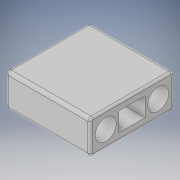
# Autodesk Inventor part: Y_Slider_Part_mit_Schrittmotor
Saved by Autodesk Inventor 2019 (Build 230136000, 136)
## iProperties
Created: 2018-08-19
Part Number: Y_Slider_Part_mit_Schrittmotor
Material: Generic
Document SubType Name: Modeling
Designer: Julia
Density: 1 g/cm^3
Appearance: Default
Author: Julia
Autodesk Inventor part; units mm, degrees
ref_plane "YZ Plane" through (0, 0, 0) normal (1, 0, 0) x (0, 1, 0)
ref_plane "XZ Plane" through (0, 0, 0) normal (0, 1, 0) x (-1, 0, 0)
ref_plane "XY Plane" through (0, 0, 0) normal (0, 0, 1) x (1, 0, 0)
sketch "Sketch1" plane through (0, 0, 0) normal (0, 1, 0) x (-1, 0, 0)
  line L0 (40, 40) -> (-40, 40)
  line L1 (-40, 40) -> (-40, -40)
  line L2 (-40, -40) -> (40, -40)
  line L3 (40, -40) -> (40, 40)
  point P0 (0, 0)
  point P1 (40, 0)
  point P2 (0, 40)
  dimension "d0" = 80
  dimension "d1" = 80
  constraints: 8 end point, 2 midpoint, 2 parallel, 1 horizontal, 1 horizontal alignment, 1 perpendicular, 1 vertical alignment
  measures "d0" distance of L2.end L0.start
  measures "d1" distance of L1.end L2.end
extrude "Extrusion1" add sketch "Sketch1" along normal blind 32
sketch "Sketch27" plane through (-40, 0, 40) normal (0, 0, 1) x (1, 0, 0)
  line L0 (20, 27) -> (60, 27)
  line L1 (60, 27) -> (60, 5)
  line L2 (60, 5) -> (20, 5)
  line L3 (20, 5) -> (20, 27)
  line L4 (0, 0) -> (80, 0) projected
  line L5 (0, 32) -> (80, 32) projected
  line L6 (0, 0) -> (0, 32) projected
  line L7 (80, 0) -> (80, 32) projected
  point P0 (40, 0)
  dimension "d171" = 5
  dimension "d172" = 5
  dimension "d173" = 20
  dimension "d174" = 20
  constraints: 8 end point, 2 parallel, 1 horizontal, 1 perpendicular
  measures "d171" distance between parallel lines of L4 L2
  measures "d172" distance between parallel lines of L5 L0
  measures "d173" distance between parallel lines of L6 L3
  measures "d174" distance between parallel lines of L7 L1
extrude "Extrusion21" cut sketch "Sketch27" against normal up to next contours L0 L1 L2 L3
sketch "Sketch28" plane through (-40, 0, -40) normal (-1, 0, 0) x (0, 0, 1)
  line L0 (0, 0) -> (0, 32) projected
  point P0 (40, 0)
  point P1 (15, 16)
  point P2 (65, 16)
  point P3 (0, 16)
  point P4 (0, 16)
  dimension "d177" = 25
  dimension "d178" = 25
  constraints: 2 horizontal alignment, 2 midpoint
  measures "d177" horizontal distance of point (40, 0) point (15, 16)
  measures "d178" horizontal distance of point (65, 16) point (40, 0)
hole "Hole8" at (-40, 16, -25) at (-40, 16, 25) direction (1, 0, 0) diameter 20 end through all
sketch "Sketch29" plane through (-40, 0, -40) normal (-1, 0, 0) x (0, 0, 1)
  line L0 (52.5, 25) -> (27.5, 25)
  line L1 (27.5, 25) -> (27.5, 7)
  line L2 (27.5, 7) -> (52.5, 7)
  line L3 (52.5, 7) -> (52.5, 25)
  line L4 (0, 32) -> (80, 32) projected
  line L5 (0, 0) -> (80, 0) projected
  point P0 (40, 0)
  point P1 (40, 7)
  point P2 (40, 0)
  dimension "d186" = 7
  dimension "d187" = 7
  dimension "d188" = 25
  constraints: 8 end point, 2 midpoint, 2 parallel, 1 horizontal, 1 perpendicular, 1 vertical alignment
  measures "d186" distance between parallel lines of L0 L4
  measures "d187" distance between parallel lines of L5 L2
  measures "d188" distance of L1.end L2.end
extrude "Extrusion22" cut sketch "Sketch29" against normal through all
extrude "Extrusion23" add sketch "Sketch27" against normal blind 4 contours L0 L1 L2 L3
sketch "Sketch30" plane through (40, 0, -40) normal (0, 0, -1) x (-1, 0, 0)
  line L0 (20, 27) -> (60, 27) projected
  line L1 (60, 5) -> (20, 5)
  line L2 (20, 5) -> (20, 27)
  line L3 (20, 27) -> (60, 27)
  line L4 (60, 27) -> (60, 5)
  point P0 (40, 0)
  constraints: 8 end point, 2 parallel, 1 horizontal, 1 perpendicular
extrude "Extrusion24" add sketch "Sketch30" against normal blind 4
fillet "Fillet23" radius 11 4 edges at (0, 5, -36) (0, 27, -36) (0, 27, 36) (0, 5, 36)
fillet "Fillet24" radius 3 4 edges at (0, 32, 40) (0, 0, 40) (0, 32, -40) (0, 0, -40)
fillet "Fillet25" radius 2 16 edges at (40, 31.1213, -39.1213) (40, 16, -40) (40, 0.8787, -39.1213) (40, 0, 0) (40, 0.8787, 39.1213) (40, 16, 40) (40, 31.1213, 39.1213) (40, 32, 0) (-40, 31.1213, 39.1213) (-40, 16, 40) (-40, 0.8787, 39.1213) (-40, 0, 0) (-40, 0.8787, -39.1213) (-40, 16, -40) (-40, 31.1213, -39.1213) (-40, 32, 0)
body "Solid1"
